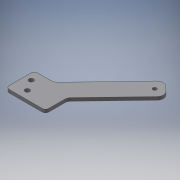
# Autodesk Inventor part: BlæserMount
Saved by Autodesk Inventor 2016 SP1 (Build 200210100, 210)
## iProperties
Created: 2015-12-22
Part Number: BlæserMount
Material: Generic
Document SubType Name: Modeling
Designer: PowerStation9000
Density: 1 g/cm^3
Appearance: Default
Author: PowerStation9000
Autodesk Inventor part; units mm, degrees
ref_plane "YZ Plane" through (0, 0, 0) normal (1, 0, 0) x (0, 1, 0)
ref_plane "XZ Plane" through (0, 0, 0) normal (0, 1, 0) x (-1, 0, 0)
ref_plane "XY Plane" through (0, 0, 0) normal (0, 0, 1) x (1, 0, 0)
sketch "Sketch1" plane through (0, 0, 0) normal (0, 0, 1) x (1, 0, 0)
  line L0 (18.5786, 18.746) -> (17.0917, 17.2136) construction
  arc A0 (17.9845, 16.2868) -> (17.0917, 17.2136) centre (-2.1377, -2.2032) ccw construction
  line L1 (17.9845, 16.2868) -> (20.1624, 18.5314) construction
  arc A1 (18.5786, 18.746) -> (20.1624, 18.5314) centre (19.5791, 20.1786) ccw construction
  arc A2 (-17.1863, -18.1767) -> (-16.167, -18.9622) centre (0, 3.0698) ccw construction
  line L2 (-18.546, -19.8229) -> (-17.1863, -18.1767) construction
  arc A3 (-18.1587, -21.3736) -> (-18.546, -19.8229) centre (-19.86, -20.9748) ccw construction
  line L3 (-18.1587, -21.3736) -> (-16.167, -18.9622) construction
  circle A4 centre (19.5791, 20.1786) radius 1.1883 construction
  arc A5 (16.6904, 17.6029) -> (15.7371, 18.4674) centre (-2.1377, -2.2032) ccw construction
  line L4 (18.1773, 19.1353) -> (16.6904, 17.6029) construction
  arc A6 (17.9151, 20.712) -> (18.1773, 19.1353) centre (19.5791, 20.1786) ccw construction
  line L5 (17.9151, 20.712) -> (15.7371, 18.4674) construction
  arc A7 (-18.5813, -16.968) -> (-17.6174, -17.8206) centre (0, 3.0698) ccw construction
  line L6 (-18.5813, -16.968) -> (-20.5731, -19.3794) construction
  arc A8 (-18.9771, -19.4668) -> (-20.5731, -19.3794) centre (-19.86, -20.9748) ccw construction
  line L7 (-18.9771, -19.4668) -> (-17.6174, -17.8206) construction
  circle A9 centre (-19.86, -20.9748) radius 1.1883 construction
  line L8 (-16.3337, 25.9034) -> (-16.8518, 26.1012) construction
  line L9 (-16.3337, 26.3055) -> (-16.3337, 25.9034) construction
  line L10 (-16.8518, 26.1012) -> (-16.3337, 26.3055) construction
  line L11 (-19.0249, 26.6328) -> (-15.9448, 26.6328) construction
  line L12 (-19.0249, 18.2452) -> (-19.0249, 26.6328) construction
  line L13 (-14.5515, 18.2452) -> (-19.0249, 18.2452) construction
  line L14 (-14.5515, 26.6328) -> (-14.5515, 18.2452) construction
  line L15 (-15.8844, 26.6328) -> (-14.5515, 26.6328) construction
  line L16 (-15.8844, 26.2285) -> (-15.8844, 26.6328) construction
  line L17 (-15.9443, 26.2285) -> (-15.8844, 26.2285) construction
  line L18 (-15.9443, 26.2676) -> (-15.9443, 26.2285) construction
  spline S0 degree 3 poles (-16.0393, 26.4068) (-16.0329, 26.4063) (-16.0204, 26.4054) (-16.0023, 26.3984) (-15.986, 26.3869) (-15.9714, 26.3711) (-15.9588, 26.3512) (-15.9505, 26.3267) (-15.9449, 26.2985) (-15.9445, 26.2783) (-15.9443, 26.2676) knots 0 0 0 0 0.101714 0.200319 0.305072 0.417926 0.542764 0.677988 0.829039 1 1 1 1 construction
  spline S1 degree 3 poles (-16.1301, 26.3857) (-16.1211, 26.3889) (-16.1041, 26.3949) (-16.0799, 26.4013) (-16.0586, 26.4058) (-16.0454, 26.4065) (-16.0393, 26.4068) knots 0 0 0 0 0.306023 0.575345 0.804378 1 1 1 1 construction
  line L19 (-16.2738, 26.3291) -> (-16.1301, 26.3857) construction
  line L20 (-16.2738, 25.8805) -> (-16.2738, 26.3291) construction
  line L21 (-16.0234, 25.7848) -> (-16.2738, 25.8805) construction
  spline S2 degree 3 poles (-15.9946, 25.7789) (-15.9993, 25.7792) (-16.0092, 25.7797) (-16.0185, 25.7831) (-16.0234, 25.7848) knots 0 0 0 0 0.478178 1 1 1 1 construction
  spline S3 degree 3 poles (-15.9602, 25.8) (-15.9622, 25.7968) (-15.9659, 25.7907) (-15.9741, 25.7836) (-15.984, 25.7798) (-15.991, 25.7792) (-15.9946, 25.7789) knots 0 0 0 0 0.261211 0.507299 0.74454 1 1 1 1 construction
  spline S4 degree 3 poles (-15.9443, 25.9058) (-15.9444, 25.8942) (-15.9446, 25.8729) (-15.9477, 25.8436) (-15.9519, 25.8195) (-15.9576, 25.806) (-15.9602, 25.8) knots 0 0 0 0 0.321536 0.594469 0.818506 1 1 1 1 construction
  line L22 (-15.9443, 25.9439) -> (-15.9443, 25.9058) construction
  line L23 (-15.8844, 25.9439) -> (-15.9443, 25.9439) construction
  line L24 (-15.8844, 25.4647) -> (-15.8844, 25.9439) construction
  line L25 (-15.9443, 25.4647) -> (-15.8844, 25.4647) construction
  line L26 (-15.9443, 25.5009) -> (-15.9443, 25.4647) construction
  spline S5 degree 3 poles (-16.0098, 25.6044) (-16.0046, 25.6021) (-15.9945, 25.5977) (-15.9809, 25.5889) (-15.9695, 25.5783) (-15.9603, 25.5659) (-15.9528, 25.5521) (-15.9478, 25.5365) (-15.9447, 25.5192) (-15.9444, 25.5072) (-15.9443, 25.5009) knots 0 0 0 0 0.12992 0.250999 0.368228 0.484041 0.601216 0.725171 0.857283 1 1 1 1 construction
  line L27 (-17.0675, 26.0083) -> (-16.0098, 25.6044) construction
  line L28 (-17.0675, 26.0792) -> (-17.0675, 26.0083) construction
  line L29 (-16.088, 26.4655) -> (-17.0675, 26.0792) construction
  spline S6 degree 3 poles (-15.9448, 26.6343) (-15.945, 26.6279) (-15.9461, 26.6118) (-15.9509, 26.5869) (-15.9601, 26.561) (-15.9738, 26.5381) (-15.993, 26.5177) (-16.0187, 26.4991) (-16.0507, 26.4811) (-16.075, 26.471) (-16.088, 26.4655) knots 0.053864 0.053864 0.053864 0.053864 0.129499 0.246974 0.354967 0.455939 0.562557 0.68682 0.832183 1 1 1 1 construction
  line L30 (-21.4293, 26.6328) -> (-21.4293, 9.8576) construction
  line L31 (-24.6726, 26.6328) -> (-21.4293, 26.6328) construction
  line L32 (-24.6726, 9.8576) -> (-24.6726, 26.6328) construction
  line L33 (-21.4293, 9.8576) -> (-24.6726, 9.8576) construction
  circle A10 centre (0, 0) radius 16.7753 construction
  line L34 (10.0608, 22.0117) -> (10.6373, 22.5863) construction
  arc A11 (15.7973, 19.3323) -> (10.6373, 22.5863) centre (0, 0) ccw construction
  line L35 (18.0541, 21.6583) -> (15.7973, 19.3323) construction
  arc A12 (21.1041, 18.6989) -> (18.0541, 21.6583) centre (19.5791, 20.1786) ccw construction
  line L36 (21.1041, 18.6989) -> (18.3133, 15.8226) construction
  arc A13 (0, -24.2019) -> (18.3133, 15.8226) centre (0, 0) ccw construction
  arc A14 (-14.8516, -19.8033) -> (0, -24.2019) centre (0, 3.0698) ccw construction
  ellipse E0 centre (-15.4609, -20.7415) end of major axis (-14.7484, -19.879) minor radius 1.1184 (-14.8516, -19.8033) -> (-16.3232, -20.0293) ccw construction
  line L37 (-16.3232, -20.0293) -> (-18.2218, -22.328) construction
  arc A15 (-21.4983, -19.6216) -> (-18.2218, -22.328) centre (-19.86, -20.9748) ccw construction
  line L38 (-21.4983, -19.6216) -> (-19.5997, -17.323) construction
  ellipse E1 centre (-20.462, -16.6108) end of major axis (-19.7495, -15.7482) minor radius 1.1184 (-19.5997, -17.323) -> (-19.6557, -15.8352) ccw construction
  arc A16 (-27.2594, 2.2506) -> (-19.6557, -15.8352) centre (0, 3.0698) ccw construction
  line L39 (-28.0761, 29.4287) -> (-27.2594, 2.2506) construction
  line L40 (-27.5723, 29.4287) -> (-28.0761, 29.4287) construction
  line L41 (-27.5723, 29.4287) -> (-26.756, 2.2658) construction
  arc A17 (-26.756, 2.2658) -> (0, -23.6983) centre (0, 3.0698) ccw construction
  arc A18 (0, -23.6983) -> (14.9112, 18.4191) centre (0, 0) ccw construction
  line L42 (14.9112, 18.4191) -> (14.8982, 18.4058) construction
  arc A19 (0, -23.6797) -> (14.8982, 18.4058) centre (0, 0) ccw construction
  arc A20 (-26.7375, 2.2663) -> (0, -23.6797) centre (0, 3.0698) ccw construction
  line L43 (-26.7375, 2.2663) -> (-27.5537, 29.4287) construction
  line L44 (-27.5537, 29.4287) -> (4.0735, 29.4287) construction
  line L45 (4.0735, 29.4287) -> (4.0735, 23.5758) construction
  spline S7 degree 3 poles (4.0735, 23.5758) (4.0735, 23.5061) (4.0979, 23.4388) (4.1866, 23.332) (4.2486, 23.2956) (4.317, 23.2829) knots 0 0 0 0 0.5 0.5 1 1 1 1 construction
  arc A21 (9.4913, 21.6944) -> (4.317, 23.2829) centre (0, 0) ccw construction
  arc A22 (9.4913, 21.6944) -> (9.5899, 21.6712) centre (9.6034, 21.9505) ccw construction
  arc A23 (9.5899, 21.6712) -> (4.3204, 23.3011) centre (0, 0) ccw construction
  spline S8 degree 3 poles (4.3204, 23.3011) (4.2885, 23.307) (4.2579, 23.3185) (4.2022, 23.3512) (4.1772, 23.3723) (4.1358, 23.4221) (4.1197, 23.4504) (4.0977, 23.5112) (4.092, 23.5434) (4.092, 23.5758) knots -0.069591 -0.069591 -0.069591 -0.069591 -0.052128 -0.052128 -0.034725 -0.034725 -0.017377 -0.017377 0 0 0 0 construction
  line L46 (4.092, 23.5758) -> (4.092, 29.4287) construction
  line L47 (5.0431, 29.4287) -> (4.092, 29.4287) construction
  line L48 (5.0431, 24.3398) -> (5.0431, 29.4287) construction
  ellipse E2 centre (5.8822, 24.3403) end of major axis (5.2221, 23.8221) minor radius 0.8388 (5.0431, 24.3398) -> (5.6847, 23.5248) ccw construction
  arc A24 (10.0608, 22.0117) -> (5.6847, 23.5248) centre (0, 0) ccw construction
  line L49 (-2.1211, -11.1365) -> (24.6029, 16.7491)
  line L50 (24.4826, 22.4047) -> (21.5947, 25.1723)
  line L51 (-28.2332, -10.1365) -> (-28.2332, -24.1365)
  line L52 (19.5791, 20.1786) -> (-19.86, -20.9748) construction
  line L53 (-28.2332, -20.9748) -> (-11.1999, -20.9748) construction
  arc A25 (24.6029, 16.7491) -> (24.4826, 22.4047) centre (21.715, 19.5168) ccw
  arc A26 (21.5947, 25.1723) -> (15.9391, 25.052) centre (18.8271, 22.2844) ccw
  arc A27 (-2.1211, -11.1365) -> (-3.2332, -13.9041) centre (0.7668, -13.9041) ccw
  circle A28 centre (19.5791, 20.1786) radius 1.1883
  circle A29 centre (-24.2332, -14.1365) radius 1.5
  line L54 (-17.5739, -8.1365) -> (-26.2332, -8.1365)
  line L55 (15.9391, 25.052) -> (-14.6859, -6.9041)
  arc A30 (-17.5739, -8.1365) -> (-14.6859, -6.9041) centre (-17.5739, -4.1365) ccw
  arc A31 (-26.2332, -8.1365) -> (-28.2332, -10.1365) centre (-26.2332, -10.1365) ccw
  circle A32 centre (-19.86, -20.9748) radius 1.5
  line L56 (-3.2332, -13.9041) -> (-3.2332, -24.1365)
  line L57 (-5.2332, -26.1365) -> (-26.2332, -26.1365)
  arc A33 (-28.2332, -24.1365) -> (-26.2332, -26.1365) centre (-26.2332, -24.1365) ccw
  arc A34 (-5.2332, -26.1365) -> (-3.2332, -24.1365) centre (-5.2332, -24.1365) ccw
  point P0 (0, 0)
  point P1 (-3.2332, -12.2969)
  dimension "d0" = 6
  dimension "d2" = 5
  dimension "d7" = 4
  dimension "d11" = 3
  dimension "d15" = 4
  dimension "d16" = 6
  dimension "d17" = 4
  dimension "d18" = 2
  dimension "d19" = 38.6236
  dimension "d23" = 3
  dimension "d25" = 6
  dimension "d26" = 18
  dimension "d27" = 15
  dimension "d28" = 25
  dimension "d29" = 2
  constraints: 18 end point, 14 point on circle, 14 tangent, 10 centre point, 4 equal radius, 3 perpendicular, 3 point on line, 2 coincident, 1 horizontal, 1 parallel, 1 vertical, 3 other
  measures "d0" distance between parallel lines of L52 L49
  measures "d2" distance from line of A4.centre L50
  measures "d7" radius of A25
  measures "d11" diameter of A29
  measures "d15" distance from line of L51 A29.centre
  measures "d16" distance between parallel lines of L52 L55
  measures "d17" radius of A30
  measures "d18" radius of A31
  measures "d19" distance of L49.start L49.end
  measures "d23" diameter of A32
  measures "d25" distance from line of L54 A29.centre
  measures "d26" distance between parallel lines of L57 L54
  measures "d27" distance from line of L57 L49.start
  measures "d28" distance between parallel lines of L51 L56
  measures "d29" radius of A33
extrude "Extrusion1" add sketch "Sketch1" along normal blind 2
equation "\"d11\" = d23"
equation "\"d16\" = d0"
equation "\"d1\" = d0"
body "Solid1"
